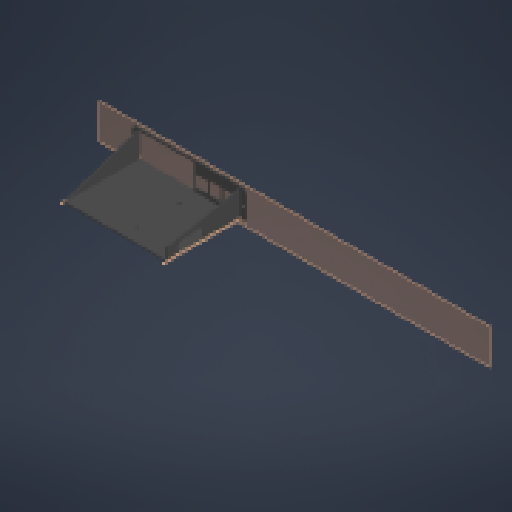
# Autodesk Inventor part: RPI_HOUSING2
Saved by Autodesk Inventor 2026.2 (Build 302298010, 298A)
## iProperties
Created: 2026-03-25
Part Number: RPI_HOUSING2
Material: Rubber, Silicone
Document SubType Name: Modeling
Designer: usr
Density: 1.25 g/cm^3
Appearance: Rubber - Black
Author: usr
Autodesk Inventor part; units mm, degrees
ref_plane "YZ Plane" through (0, 0, 0) normal (1, 0, 0) x (0, 1, 0)
ref_plane "XZ Plane" through (0, 0, 0) normal (0, 1, 0) x (-1, 0, 0)
ref_plane "XY Plane" through (0, 0, 0) normal (0, 0, 1) x (1, 0, 0)
ref_plane "Work Plane1" through (0, 0, 108.3756) normal (0, 0, 1) x (1, 0, 0)
sketch "Sketch1" plane through (0, 0, 108.3756) normal (0, 0, 1) x (1, 0, 0)
  line L0 (-71.3, 18) -> (-71.3, -18) projected
  line L1 (-71.3, -18) -> (-211.3, -18) projected
  line L2 (-211.3, -18) -> (-211.3, 18) projected
  line L3 (-211.3, 18) -> (-71.3, 18) projected
  line L4 (71.3003, -18) -> (71.3003, 18) projected
  line L5 (71.3003, 18) -> (211.3003, 18) projected
  line L6 (211.3003, 18) -> (211.3003, -18) projected
  line L7 (211.3003, -18) -> (71.3003, -18) projected
  line L8 (-241.3, 22) -> (241.3, 22) projected
  line L9 (-241.3, -22) -> (-241.3, 22) projected
  line L10 (241.3, -22) -> (-241.3, -22) projected
  line L11 (241.3, 22) -> (241.3, -22) projected
  circle A0 centre (-232.5, -15.875) radius 3.5 projected
  circle A1 centre (-232.5, 15.875) radius 3.5 projected
  circle A2 centre (232.5, -15.875) radius 3.5 projected
  circle A3 centre (232.5, 15.875) radius 3.5 projected
  line L12 (-219.3, 10) -> (-219.3, -10)
  line L13 (-63.3, 10) -> (-63.3, -10)
  arc A4 (-211.3, 18) -> (-219.3, 10) centre (-211.3, 10) ccw
  arc A5 (-219.3, -10) -> (-211.3, -18) centre (-211.3, -10) ccw
  arc A6 (-63.3, 10) -> (-71.3, 18) centre (-71.3, 10) ccw
  arc A7 (-71.3, -18) -> (-63.3, -10) centre (-71.3, -10) ccw
  line L14 (-211.3, 18) -> (-71.3, 18)
  line L15 (-71.3, -18) -> (-211.3, -18)
  circle A8 centre (-215.3, 0) radius 2
  circle A9 centre (-67.3, 0) radius 2
  point P0 (0, 0)
  point P1 (-63.3, 0)
  dimension "d0" = 8
  dimension "d1" = 8
  dimension "d5" = 4
  dimension "d6" = 4
  dimension "d7" = 18
  dimension "d9" = 4
  dimension "d106" = 18
  constraints: 8 end point, 8 point on circle, 8 tangent, 6 centre point, 2 vertical, 1 equal radius, 1 horizontal, 1 midpoint, 1 parallel
  measures "d0" distance between parallel lines of L0 L13
  measures "d1" distance between parallel lines of L12 L2
  measures "d5" diameter of A9
  measures "d6" distance of point (-63.3, 0) A9.centre
  measures "d7" distance from line of L1 A9.centre
  measures "d9" distance from line of L12 A8.centre
  measures "d106" distance from line of L1 A8.centre
extrude "Extrusion2" add sketch "Sketch1" along normal blind 2 contours A6 L13 A7 L0 | L0 L1 L2 L3 | L2 A5 L12 A4
ref_plane "Work Plane4" through (-211.3, -18, 108.3756) normal (0, -1, 0) x (1, 0, 0)
sketch "Sketch3" plane through (-211.3, -18, 108.3756) normal (0, -1, 0) x (1, 0, 0)
  line L0 (0, 2) -> (140, 2) projected
  line L1 (0, 2) -> (140, 2)
  line L2 (140, 2) -> (140, 102)
  line L3 (140, 102) -> (0, 102)
  line L4 (0, 102) -> (0, 2)
  point P0 (211.3, -108.3756)
  point P1 (140, 2)
  dimension "d14" = 100
  dimension "d15" = 0
  constraints: 8 end point, 2 parallel, 1 horizontal, 1 perpendicular
  measures "d14" distance of L1.end L2.end
  measures "d15" distance from line of L2 L0.end
extrude "Extrusion3" add sketch "Sketch3" against normal blind 2
ref_plane "Work Plane5" through (-71.3, -18, 210.3756) normal (1, 0, 0) x (0, 0, -1)
sketch "Sketch4" plane through (-71.3, -18, 210.3756) normal (1, 0, 0) x (0, 0, -1)
  line L0 (0, 2) -> (100, 2) projected
  line L1 (100, 2) -> (1, 2)
  line L2 (1, 2) -> (100, 36)
  line L3 (100, 36) -> (100, 2)
  point P0 (210.3756, 18)
  dimension "d19" = 99
  constraints: 6 end point, 1 perpendicular, 1 point on line
  measures "d19" distance of L0.end L1.end
extrude "Side" add sketch "Sketch4" against normal blind 2
ref_plane "Work Plane6" through (-211.3, -18, 110.3756) normal (-1, 0, 0) x (0, 0, 1)
sketch "Sketch5" plane through (-211.3, -18, 110.3756) normal (-1, 0, 0) x (0, 0, 1)
  line L0 (0, 2) -> (100, 2) projected
  line L1 (0, 2) -> (99, 2)
  line L2 (0, 36) -> (99, 2) projected
  line L3 (0, 36) -> (99, 2)
  line L4 (0, 36) -> (0, 2)
  point P0 (-110.3756, 18)
  constraints: 6 end point, 1 collinear, 1 perpendicular, 1 point on line
extrude "Extrusion5" add sketch "Sketch5" against normal blind 2
sketch "Sketch7" plane through (0, 0, 110.3756) normal (0, 0, 1) x (1, 0, 0)
  line L0 (-209.3, -16) -> (-73.3, -16) projected
  line L1 (-129.3, -16) -> (-204.3, -16)
  line L2 (-134.3, 18) -> (-209.3, 18)
  line L3 (-134.3, -18) -> (-134.3, 18)
  line L4 (-209.3, 18) -> (-209.3, -16) projected
  line L5 (-209.3, -18) -> (-134.3, -18)
  line L6 (-209.3, -18) -> (-134.3, -18)
  line L7 (-209.3, 18) -> (-134.3, 18)
  line L8 (-134.3, 18) -> (-134.3, -18)
  line L9 (-134.3, -18) -> (-209.3, -18)
  line L10 (-209.3, -18) -> (-209.3, 18)
  point P0 (0, 0)
  point P1 (-134.3, -16)
  constraints: 18 end point, 4 horizontal, 2 parallel, 1 perpendicular, 1 point on line, 1 vertical, 4 other
extrude "Extrusion7" cut sketch "Sketch7" against normal through all contours L4 L2 L3 L0
sketch "Sketch14" plane through (0, 0, 108.3756) normal (0, 0, -1) x (-1, 0, 0)
  line L0 (116.3, 4.1) -> (131.8, 4.1) projected
  line L1 (110.85, 6.1) -> (99.75, 6.1) projected
  line L2 (80.95, 6.1) -> (93.65, 6.1) projected
  line L3 (131.8, -9.2) -> (131.8, 3.9) projected
  line L4 (116.3, 3.9) -> (116.3, -9.2) projected
  line L5 (112.15, 1.24) -> (112.15, 5.24) projected
  line L6 (112.15, -7.26) -> (112.15, -3.26) projected
  line L7 (98.05, -3.56) -> (98.05, -6.96) projected
  line L8 (98.05, 4.94) -> (98.05, 1.54) projected
  line L9 (81.3, -9.4) -> (131.3, -9.4) projected
  line L10 (94.1, -2.96) -> (94.1, -6.76) projected
  line L11 (94.1, 0.7) -> (94.1, 4.5) projected
  line L12 (80.5, 0.7) -> (80.5, 4.5) projected
  line L13 (80.5, -2.96) -> (80.5, -6.76) projected
  line L14 (79.5, 7.1) -> (95.1, 7.1)
  line L15 (95.1, 7.1) -> (95.1, -10.4)
  line L16 (95.1, -10.4) -> (79.5, -10.4)
  line L17 (79.5, -10.4) -> (79.5, 7.1)
  line L18 (97.05, 7.1) -> (113.15, 7.1)
  line L19 (113.15, 7.1) -> (113.15, -10.4)
  line L20 (113.15, -10.4) -> (97.05, -10.4)
  line L21 (97.05, -10.4) -> (97.05, 7.1)
  line L22 (115.3, 5.1) -> (132.8, 5.1)
  line L23 (132.8, 5.1) -> (132.8, -10.4)
  line L24 (132.8, -10.4) -> (115.3, -10.4)
  line L25 (115.3, -10.4) -> (115.3, 5.1)
  point P0 (0, 0)
  dimension "d54" = 1
  dimension "d55" = 1
  dimension "d56" = 1
  dimension "d58" = 1
  dimension "d59" = 1
  dimension "d60" = 1
  dimension "d61" = 1
  dimension "d62" = 1
  dimension "d63" = 1
  dimension "d64" = 1
  dimension "d65" = 1
  dimension "d66" = 1
  constraints: 24 end point, 6 parallel, 3 horizontal, 3 perpendicular
  measures "d54" distance between parallel lines of L9 L24
  measures "d55" distance between parallel lines of L3 L23
  measures "d56" distance between parallel lines of L0 L22
  measures "d58" distance between parallel lines of L1 L18
  measures "d59" distance between parallel lines of L19 L5
  measures "d60" distance between parallel lines of L9 L20
  measures "d61" distance between parallel lines of L9 L16
  measures "d62" distance between parallel lines of L11 L15
  measures "d63" distance between parallel lines of L2 L14
  measures "d64" distance between parallel lines of L17 L12
  measures "d65" distance between parallel lines of L7 L21
  measures "d66" distance between parallel lines of L25 L4
extrude "Extrusion12" cut sketch "Sketch14" against normal up to surface (2 mm away)
sketch "Sketch16" plane through (-211.3, -18, 108.3756) normal (0, -1, 0) x (1, 0, 0)
  circle A0 centre (80.5, 83.5) radius 1.35 projected
  circle A1 centre (129.5, 83.5) radius 1.35 projected
  circle A2 centre (80.5, 25.5) radius 1.35 projected
  circle A3 centre (129.5, 25.5) radius 1.35 projected
  circle A4 centre (129.5, 25.5) radius 2
  circle A5 centre (80.5, 25.5) radius 2
  circle A6 centre (80.5, 83.5) radius 2
  circle A7 centre (129.5, 83.5) radius 2
  point P0 (211.3, -108.3756)
  dimension "d102" = 4
  dimension "d103" = 4
  dimension "d104" = 4
  dimension "d105" = 4
  constraints: 4 centre point, 4 coincident
  measures "d102" diameter of A4
  measures "d103" diameter of A5
  measures "d104" diameter of A6
  measures "d105" diameter of A7
extrude "Extrusion14" cut sketch "Sketch16" against normal up to surface (2 mm away) contours A0 | A1 | A2 | A3 | A4 | A5 | A6 | A7
sketch "Sketch18" plane through (-211.3, -18, 108.3756) normal (0, -1, 0) x (1, 0, 0)
  circle A0 centre (129.5001, 83.5001) radius 1.2643 projected
  circle A1 centre (129.5001, 25.5001) radius 1.2643 projected
  line L0 (77.0359, 25.5) -> (78.7679, 28.5)
  line L1 (78.7679, 28.5) -> (82.2321, 28.5)
  line L2 (82.2321, 28.5) -> (83.9641, 25.5)
  line L3 (83.9641, 25.5) -> (82.2321, 22.5)
  line L4 (82.2321, 22.5) -> (78.7679, 22.5)
  line L5 (78.7679, 22.5) -> (77.0359, 25.5)
  line L6 (75.0359, 25.5) -> (77.7679, 30.2321)
  line L7 (77.7679, 30.2321) -> (83.2321, 30.2321)
  line L8 (83.2321, 30.2321) -> (85.9641, 25.5)
  line L9 (85.9641, 25.5) -> (83.2321, 20.7679)
  line L10 (83.2321, 20.7679) -> (77.7679, 20.7679)
  line L11 (77.7679, 20.7679) -> (75.0359, 25.5)
  line L12 (77.0359, 83.5) -> (78.7679, 86.5)
  line L13 (78.7679, 86.5) -> (82.2321, 86.5)
  line L14 (82.2321, 86.5) -> (83.9641, 83.5)
  line L15 (83.9641, 83.5) -> (82.2321, 80.5)
  line L16 (82.2321, 80.5) -> (78.7679, 80.5)
  line L17 (78.7679, 80.5) -> (77.0359, 83.5)
  line L18 (75.0359, 83.5) -> (77.7679, 88.2321)
  line L19 (77.7679, 88.2321) -> (83.2321, 88.2321)
  line L20 (83.2321, 88.2321) -> (85.9641, 83.5)
  line L21 (85.9641, 83.5) -> (83.2321, 78.7679)
  line L22 (83.2321, 78.7679) -> (77.7679, 78.7679)
  line L23 (77.7679, 78.7679) -> (75.0359, 83.5)
  line L24 (126.036, 83.5001) -> (127.7681, 86.5001)
  line L25 (127.7681, 86.5001) -> (131.2322, 86.5001)
  line L26 (131.2322, 86.5001) -> (132.9642, 83.5001)
  line L27 (132.9642, 83.5001) -> (131.2322, 80.5001)
  line L28 (131.2322, 80.5001) -> (127.7681, 80.5001)
  line L29 (127.7681, 80.5001) -> (126.036, 83.5001)
  line L30 (124.036, 83.5001) -> (126.7681, 88.2321)
  line L31 (126.7681, 88.2321) -> (132.2322, 88.2321)
  line L32 (132.2322, 88.2321) -> (134.9642, 83.5001)
  line L33 (134.9642, 83.5001) -> (132.2322, 78.768)
  line L34 (132.2322, 78.768) -> (126.7681, 78.768)
  line L35 (126.7681, 78.768) -> (124.036, 83.5001)
  line L36 (126.036, 25.5001) -> (127.7681, 28.5001)
  line L37 (127.7681, 28.5001) -> (131.2322, 28.5001)
  line L38 (131.2322, 28.5001) -> (132.9642, 25.5001)
  line L39 (132.9642, 25.5001) -> (131.2322, 22.5001)
  line L40 (131.2322, 22.5001) -> (127.7681, 22.5001)
  line L41 (127.7681, 22.5001) -> (126.036, 25.5001)
  line L42 (124.036, 25.5001) -> (126.7681, 30.2322)
  line L43 (126.7681, 30.2322) -> (132.2322, 30.2322)
  line L44 (132.2322, 30.2322) -> (134.9642, 25.5001)
  line L45 (134.9642, 25.5001) -> (132.2322, 20.7681)
  line L46 (132.2322, 20.7681) -> (126.7681, 20.7681)
  line L47 (126.7681, 20.7681) -> (124.036, 25.5001)
  line L48 (0, 0) -> (140, 0) projected
  circle A2 centre (80.5, 25.5) radius 2 projected
  circle A3 centre (129.5, 25.5) radius 2 projected
  circle A4 centre (80.5, 83.5) radius 2 projected
  point P0 (211.3, -108.3756)
  dimension "d91" = 6
  dimension "d92" = 2
  dimension "d93" = 6
  dimension "d94" = 2
  dimension "d95" = 6
  dimension "d96" = 2
  dimension "d97" = 6
  dimension "d99" = 2
  constraints: 96 end point, 8 coincident, 8 parallel, 104 other
  measures "d91" distance between parallel lines of L3 L0
  measures "d92" distance of L6.start L0.start
  measures "d93" distance between parallel lines of L15 L12
  measures "d94" distance of L12.start L18.start
  measures "d95" distance between parallel lines of L27 L24
  measures "d96" distance of L30.start L24.start
  measures "d97" distance between parallel lines of L39 L36
  measures "d99" distance of L42.start L36.start
extrude "Extrusion16" add sketch "Sketch18" along normal blind 2 contours L6 L7 L8 L9 L10 L11 | L18 L19 L20 L21 L22 L23 | L30 L31 L32 L33 L34 L35 | L42 L43 L44 L45 L46 L47
fillet "Fillet1" radius 1.5 2 edges at (-69.3, 0, 108.3756) (-217.3, 0, 108.3756)
sketch "Sketch19" plane through (0, 0, 108.3756) normal (0, 0, -1) x (-1, 0, 0)
  circle A0 centre (67.3, 0) radius 3.5 projected
  line L0 (79.5, 7.1) -> (95.1, 7.1) projected
  line L1 (95.1, 7.1) -> (95.1, -10.4) projected
  line L2 (95.1, -10.4) -> (79.5, -10.4) projected
  line L3 (79.5, -10.4) -> (79.5, 7.1) projected
  line L4 (132.8, -10.4) -> (115.3, -10.4) projected
  line L5 (115.3, -10.4) -> (115.3, 5.1) projected
  line L6 (115.3, 5.1) -> (132.8, 5.1) projected
  line L7 (132.8, 5.1) -> (132.8, -10.4) projected
  line L8 (97.05, -10.4) -> (97.05, 7.1) projected
  line L9 (97.05, 7.1) -> (113.15, 7.1) projected
  line L10 (113.15, 7.1) -> (113.15, -10.4) projected
  line L11 (113.15, -10.4) -> (97.05, -10.4) projected
  line L12 (209.3, 18) -> (209.3, -16) projected
  line L13 (209.3, -16) -> (134.3, -16) projected
  line L14 (134.3, -16) -> (134.3, 18) projected
  line L15 (71.3, 18) -> (134.3, 18) projected
  arc A1 (71.3, 18) -> (63.3, 10) centre (71.3, 10) ccw projected
  line L16 (63.3, -10) -> (63.3, 10) projected
  arc A2 (63.3, -10) -> (71.3, -18) centre (71.3, -10) ccw projected
  line L17 (211.3, -18) -> (71.3, -18) projected
  arc A3 (211.3, -18) -> (219.3, -10) centre (211.3, -10) ccw projected
  line L18 (219.3, 10) -> (219.3, -10) projected
  arc A4 (219.3, 10) -> (211.3, 18) centre (211.3, 10) ccw projected
  line L19 (209.3, 18) -> (211.3, 18) projected
  circle A5 centre (215.3, 0) radius 3.5 projected
  line L20 (71.3, 21) -> (211.3, 21)
  line L21 (63.3, 10) -> (63.3, 13)
  line L22 (63.3, -10) -> (63.3, -13)
  line L23 (219.3, 10) -> (219.3, 13)
  line L24 (219.3, -10) -> (219.3, -13)
  line L25 (71.3, -21) -> (211.3, -21)
  arc A6 (211.3, -21) -> (219.3, -13) centre (211.3, -13) ccw
  arc A7 (219.3, 13) -> (211.3, 21) centre (211.3, 13) ccw
  arc A8 (71.3, 21) -> (63.3, 13) centre (71.3, 13) ccw
  arc A9 (63.3, -13) -> (71.3, -21) centre (71.3, -13) ccw
  line L26 (209.3, 18) -> (134.3, 18)
  point P0 (0, 0)
  dimension "d108" = 3
  dimension "d109" = 3
  dimension "d110" = 3
  dimension "d111" = 3
  dimension "d112" = 3
  dimension "d114" = 3
  constraints: 14 end point, 9 tangent, 8 point on circle, 4 centre point, 4 vertical, 3 horizontal
  measures "d108" distance between parallel lines of L15 L20
  measures "d109" distance of L16.end L21.end
  measures "d110" distance of L16.start L22.end
  measures "d111" distance of L18.start L23.end
  measures "d112" distance of L18.end L24.end
  measures "d114" distance between parallel lines of L25 L17
extrude "Extrusion17" add sketch "Sketch19" against normal blind 2 contours L26 L15 A1 L21 A8 L20 A7 L23 A4 L19 | L24 A6 L25 A9 L22 A2 L17 A3
sketch "Sketch20" plane through (-71.3, -18, 210.3756) normal (1, 0, 0) x (0, 0, -1)
  line L0 (100, 36) -> (1, 2)
  line L1 (1, 2) -> (1, 17)
  line L2 (102, 36) -> (100, 36) projected
  line L3 (1, 17) -> (100, 36)
  point P0 (210.3756, 18)
  dimension "d117" = 15
  constraints: 6 end point, 1 vertical, 3 other
  measures "d117" distance of L0.end L1.end
extrude "Extrusion18" add sketch "Sketch20" against normal blind 2
sketch "Sketch21" plane through (-71.3, -18, 210.3756) normal (1, 0, 0) x (0, 0, -1)
  line L0 (1, 2) -> (100, 2)
  line L1 (100, 36) -> (1, 17)
  line L2 (16, 2) -> (51, 2)
  line L3 (51, 2) -> (51, 11)
  line L4 (45, 17) -> (22, 17)
  line L5 (16, 11) -> (16, 2)
  line L6 (1, 17) -> (1, 2) projected
  arc A0 (22, 17) -> (16, 11) centre (22, 11) ccw
  arc A1 (51, 11) -> (45, 17) centre (45, 11) ccw
  arc A2 (16, 7) -> (21, 2) centre (21, 7) ccw
  arc A3 (46, 2) -> (51, 7) centre (46, 7) ccw
  point P0 (210.3756, 18)
  point P1 (21, 2)
  point P2 (46, 2)
  dimension "d120" = 15
  dimension "d121" = 15
  dimension "d122" = 50
  dimension "d123" = 6
  dimension "d124" = 5
  dimension "d125" = 5
  constraints: 12 end point, 8 point on circle, 8 tangent, 5 point on line, 4 centre point, 2 horizontal, 2 parallel, 1 equal radius, 1 perpendicular, 5 other
  measures "d120" distance between parallel lines of L0 L4
  measures "d121" distance between parallel lines of L6 L5
  measures "d122" distance between parallel lines of L6 L3
  measures "d123" radius of A0
  measures "d124" radius of A2
  measures "d125" radius of A3
extrude "Extrusion19" cut sketch "Sketch21" against normal blind 2 contours A2 L5 A0 L4 A1 L3 A3 L0
body "Solid2"
